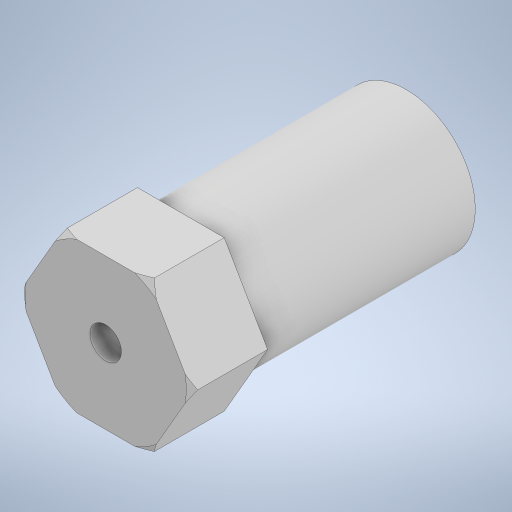
# Autodesk Inventor part: PIN
Saved by Autodesk Inventor 2024 (Build 280153000, 153)
## iProperties
Created: 2023-10-30
Part Number: PIN
Material: Generic
Document SubType Name: Modeling
Designer: jebes windows
Density: 1 g/cm^3
Appearance: Default
Author: jebes windows
## iProperties of the stored document PIN_3DPrint.ipt
Created: 2023-10-30
Part Number: PIN_3DPrint
Material: Generic
Document SubType Name: Modeling
Designer: jebes windows
Density: 1 g/cm^3
Appearance: Default
Author: jebes windows
Autodesk Inventor part; units mm, degrees
ref_plane "YZ Plane" through (0, 0, 0) normal (1, 0, 0) x (0, 1, 0)
ref_plane "XZ Plane" through (0, 0, 0) normal (0, 1, 0) x (-1, 0, 0)
ref_plane "XY Plane" through (0, 0, 0) normal (0, 0, 1) x (1, 0, 0)
sketch "Sketch7" plane through (0, 0, 0) normal (0, 1, 0) x (-1, 0, 0)
  line L0 (-3.4641, -6) -> (-6.9282, 0)
  line L1 (-6.9282, 0) -> (-3.4641, 6)
  line L2 (-3.4641, 6) -> (3.4641, 6)
  line L3 (3.4641, 6) -> (6.9282, 0)
  line L4 (6.9282, 0) -> (3.4641, -6)
  line L5 (3.4641, -6) -> (-3.4641, -6)
  point P0 (0, 0)
  point P1 (0, 0)
  point P2 (0, -6)
  dimension "d24" = 12
  constraints: 12 end point, 1 coincident, 1 horizontal alignment, 1 midpoint, 13 other
  measures "d24" distance from line of point (0, -6) L2
extrude "Extrusion6" add sketch "Sketch7" along normal blind 6
sketch "Sketch8" plane through (0, 6, 0) normal (0, 1, 0) x (1, 0, 0)
  circle A0 centre (0, 0) radius 5.5
  circle A1 centre (0, 0) radius 2.55
  line L0 (-0.0689, 2.5491) -> (-0.0689, -1.9509)
  line L1 (-0.0689, -1.9509) -> (-1.6421, -1.9509)
  line L2 (-0.0689, -1.9509) -> (1.6421, -1.9509)
  dimension "d27" = 11
  dimension "d28" = 5.1
  dimension "d29" = 4.5
  dimension "d30" = 1.5732
  constraints: 6 end point, 3 point on circle, 2 centre point, 2 coincident, 1 perpendicular, 1 point on line, 1 vertical
  measures "d27" diameter of A0
  measures "d28" diameter of A1
  measures "d29" distance of L0.start L0.end
  measures "d30" distance of L0.end L1.end
extrude "Extrusion7" add sketch "Sketch8" along normal blind 18 contours A0 | A1 L1 L2
sketch "Sketch9" plane through (0, 0, 0) normal (0, 0, 1) x (1, 0, 0)
  line L0 (6.9282, 0) -> (3.4641, 0) projected
  line L1 (6.9282, 0) -> (6.4282, 0)
  line L2 (6.8032, 0.3147) -> (6.4282, 0)
  line L3 (6.9282, 0) -> (6.9282, 0.3868)
  line L4 (0, -4.8) -> (0, 28.8) projected
  line L5 (6.8032, 0.3147) -> (6.9282, 0.4195)
  line L6 (6.9282, 0.4195) -> (6.9282, 0.3868)
  point P0 (0, 0)
  dimension "d33" = 0.5
  dimension "d35" = 40
  dimension "d39" = 0.125
  dimension "d40" = 0.1049
  constraints: 10 end point, 2 vertical, 1 point on line
  measures "d33" distance of L0.start L1.end
  measures "d35" angle of L2 L0
  measures "d39" horizontal distance of L2.start L5.end
  measures "d40" vertical distance of L2.start L5.end
revolve "Revolution1" cut sketch "Sketch9" angle 360 about axis through (0, -10, 0) along (0, 1, 0)
chamfer "Chamfer3" distance 1 angle 45 2 edges at (0, 24, -2.55) (0, 24, 1.9509)
sketch "Sketch10" plane through (0, 0, 0) normal (0, -1, 0) x (1, 0, 0)
  circle A0 centre (0, 0) radius 1.25
  dimension "d44" = 2.5
  constraints: 1 centre point, 1 coincident
  measures "d44" diameter of A0
extrude "Extrusion8" cut sketch "Sketch10" against normal through all
body "Solid2"
